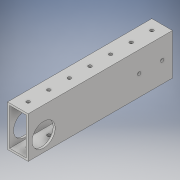
# Autodesk Inventor part: Diag_intake_hanger
Saved by Autodesk Inventor 2018 (Build 220112000, 112)
## iProperties
Created: 2018-09-07
Part Number: Diag_intake_hanger
Material: Generic
Document SubType Name: Modeling
Designer: baoan
Density: 1 g/cm^3
Appearance: Default
Author: baoan
Autodesk Inventor part; units mm, degrees
ref_plane "YZ Plane" through (0, 0, 0) normal (1, 0, 0) x (0, 1, 0)
ref_plane "XZ Plane" through (0, 0, 0) normal (0, 1, 0) x (-1, 0, 0)
ref_plane "XY Plane" through (0, 0, 0) normal (0, 0, 1) x (1, 0, 0)
sketch "Sketch1" plane through (0, 0, 0) normal (0, 0, 1) x (1, 0, 0)
  line L0 (-12.7, -25.4) -> (12.7, -25.4)
  line L1 (12.7, -25.4) -> (12.7, 25.4)
  line L2 (12.7, 25.4) -> (-12.7, 25.4)
  line L3 (-12.7, 25.4) -> (-12.7, -25.4)
  line L4 (-12.7, -25.4) -> (12.7, 25.4) construction
  line L5 (12.7, -25.4) -> (-12.7, 25.4) construction
  line L6 (-10.16, -22.86) -> (10.16, -22.86)
  line L7 (10.16, -22.86) -> (10.16, 22.86)
  line L8 (10.16, 22.86) -> (-10.16, 22.86)
  line L9 (-10.16, 22.86) -> (-10.16, -22.86)
  line L10 (-10.16, -22.86) -> (10.16, 22.86) construction
  line L11 (10.16, -22.86) -> (-10.16, 22.86) construction
  point P0 (0, 0)
  dimension "d0" = 25.4
  dimension "d1" = 50.8
  dimension "d2" = 20.32
  dimension "d3" = 45.72
  constraints: 24 end point, 4 midpoint, 4 parallel, 2 horizontal, 2 perpendicular
  measures "d0" distance of L2.end L1.end
  measures "d1" distance of L1.end L0.end
  measures "d2" distance of L8.end L7.end
  measures "d3" distance of L7.end L6.end
extrude "Extrusion1" add sketch "Sketch1" along normal mid plane 177.8
sketch "Sketch2" plane through (-12.7, 25.4, 88.9) normal (0, 1, 0) x (1, 0, 0)
  line L0 (0, 177.8) -> (0, 0) projected
  line L1 (25.4, 0) -> (0, 0) projected
  point P0 (12.7, 88.9)
  point P1 (12.7, 12.7)
  dimension "d6" = 12.7
  dimension "d7" = 12.7
  measures "d6" distance from line of L0 point (12.7, 12.7)
  measures "d7" distance from line of L1 point (12.7, 12.7)
hole "Hole1" at (0, 25.4, 76.2) direction (0, -1, 0) diameter 4.1402 end through all
pattern_linear "Rectangular Pattern1" count 7 spacing 25.4 along (0, 0, -1) of "Hole1"
sketch "Sketch3" plane through (12.7, -25.4, 88.9) normal (1, 0, 0) x (0, 0, -1)
  line L0 (0, 0) -> (0, 50.8) projected
  line L1 (177.8, 0) -> (0, 0) projected
  line L2 (177.8, 50.8) -> (177.8, 0) projected
  circle A0 centre (19.05, 19.05) radius 14.2748
  line L3 (177.8, 50.8) -> (0, 50.8) projected
  circle A1 centre (136.7019, 25.4) radius 2.0701
  circle A2 centre (165.1, 25.4) radius 2.0701
  point P0 (88.9, 25.4)
  dimension "d19" = 19.05
  dimension "d28" = 19.05
  dimension "d32" = 28.5496
  dimension "d35" = 25.4
  dimension "d36" = 12.7
  dimension "d37" = 28.3981
  dimension "d38" = 4.1402
  dimension "d39" = 4.1402
  constraints: 3 centre point, 3 coincident, 1 horizontal alignment
  measures "d19" distance from line of L0 point (19.05, 19.05)
  measures "d28" distance from line of L1 point (19.05, 19.05)
  measures "d32" diameter of A0
  measures "d35" distance from line of L3 point (165.1, 25.4)
  measures "d36" distance from line of L2 point (165.1, 25.4)
  measures "d37" distance of point (165.1, 25.4) point (136.702, 25.4)
  measures "d38" diameter of A1
  measures "d39" diameter of A2
extrude "Extrusion2" cut sketch "Sketch3" against normal through all contours A0 | A1 | A2
body "Solid1"
